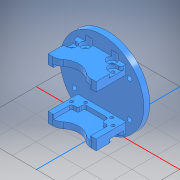
# Autodesk Inventor part: 000.005.005.001 - Основание
Saved by Autodesk Inventor 2022 (Build 260153000, 153)
## iProperties
Created: 2022-12-19
Part Number: 000.005.005.001 - Основание
Material: Пластик АБС
Document SubType Name: Modeling
Designer: Ivan Petrov
Density: 1.06 g/cm^3
Appearance: Голубой
Author: Ivan Petrov
Autodesk Inventor part; units mm, degrees
ref_plane "YZ Plane" through (0, 0, 0) normal (1, 0, 0) x (0, 1, 0)
ref_plane "XZ Plane" through (0, 0, 0) normal (0, 1, 0) x (-1, 0, 0)
ref_plane "XY Plane" through (0, 0, 0) normal (0, 0, 1) x (1, 0, 0)
sketch "Эскиз1" plane through (0, 0, 0) normal (0, 0, 1) x (1, 0, 0)
  circle A0 centre (0, 0) radius 35
  dimension "d7" = 70
  constraints: 1 centre point
  measures "d7" diameter of A0
extrude "Выдавливание1" add sketch "Эскиз1" along normal blind 5
sketch "Эскиз2" plane through (0, 0, 5) normal (0, 0, 1) x (1, 0, 0)
  circle A0 centre (-23, 15) radius 2
  point P0 (0, 0)
  dimension "d4" = 4
  dimension "d5" = 15
  dimension "d6" = 23
  constraints: 1 centre point
  measures "d4" diameter of A0
  measures "d5" vertical distance of A0.centre point (0, 0)
  measures "d6" horizontal distance of point (0, 0) A0.centre
extrude "Выдавливание2" cut sketch "Эскиз2" against normal through all
mirror "Зеркальное отражение1" about plane through (0, 0, 0) normal (0, 1, 0) of "Выдавливание2"
mirror "Зеркальное отражение2" about plane through (0, 0, 0) normal (1, 0, 0) of "Выдавливание2", "Зеркальное отражение1"
sketch "Эскиз9" plane through (0, 0, 5) normal (0, 0, 1) x (1, 0, 0)
  line L0 (20.1, 16) -> (20.1, 13.5) projected
  line L1 (-20.1, 16) -> (-20.1, 13.5) projected
  line L2 (20.1, 16) -> (-20.1, 16)
  line L3 (-20.1, 16) -> (-20.1, 18.6)
  line L4 (-20.1, 18.6) -> (20.1, 18.6)
  line L5 (20.1, 18.6) -> (20.1, 16)
  line L6 (-13, 18.6) -> (13, 18.6)
  point P0 (0, 0)
  constraints: 10 end point, 2 horizontal, 2 parallel, 1 perpendicular, 1 point on line, 2 other
extrude "Выдавливание8" add sketch "Эскиз9" along normal blind 25
sketch "Эскиз10" plane through (0, 0, 5) normal (0, 0, 1) x (1, 0, 0)
  line L0 (20.1, -15.5) -> (20.1, -18) projected
  line L1 (-20.1, -15.5) -> (-20.1, -18) projected
  line L2 (20.1, -18) -> (-20.1, -18)
  line L3 (-20.1, -18) -> (-20.1, -21.5)
  line L4 (-20.1, -21.5) -> (20.1, -21.5)
  line L5 (20.1, -21.5) -> (20.1, -18)
  line L6 (7.6826, -21.5) -> (-7.6826, -21.5) projected
  point P0 (0, 0)
  constraints: 8 end point, 2 parallel, 1 horizontal, 1 perpendicular, 1 point on line
extrude "Выдавливание9" add sketch "Эскиз10" along normal blind 25
sketch "Эскиз11" plane through (-20.1, 18.6, 5) normal (0, 1, 0) x (1, 0, 0)
  arc A0 (0, -52.6766) -> (0.5192, -54.3636) centre (3, -52.6766) ccw
  line L0 (0.5192, -54.3636) -> (4.5047, -60.2246)
  arc A1 (4.5047, -60.2246) -> (6.1586, -61.1) centre (6.1586, -59.1) ccw
  line L1 (7.1, -61.1) -> (6.1586, -61.1)
  arc A2 (5.6, -59.6) -> (7.1, -61.1) centre (7.1, -59.6) ccw
  line L2 (5.6, -6.6) -> (5.6, -59.6)
  arc A3 (6.6, -5.6) -> (5.6, -6.6) centre (6.6, -6.6) ccw
  line L3 (33.6, -5.6) -> (6.6, -5.6)
  arc A4 (34.6, -6.6) -> (33.6, -5.6) centre (33.6, -6.6) ccw
  line L4 (34.6, -59.6) -> (34.6, -6.6)
  arc A5 (33.1, -61.1) -> (34.6, -59.6) centre (33.1, -59.6) ccw
  line L5 (34.0414, -61.1) -> (33.1, -61.1)
  arc A6 (34.0414, -61.1) -> (35.6953, -60.2246) centre (34.0414, -59.1) ccw
  line L6 (35.6953, -60.2246) -> (39.6808, -54.3636)
  arc A7 (39.6808, -54.3636) -> (40.2, -52.6766) centre (37.2, -52.6766) ccw
  line L7 (40.2, -52.6766) -> (40.2, -8.4234)
  arc A8 (40.2, -8.4234) -> (39.6808, -6.7364) centre (37.2, -8.4234) ccw
  line L8 (39.6808, -6.7364) -> (35.9929, -1.3131)
  arc A9 (35.9929, -1.3131) -> (33.5121, 0) centre (33.5121, -3) ccw
  line L9 (33.5121, 0) -> (6.6879, 0)
  arc A10 (6.6879, 0) -> (4.2071, -1.3131) centre (6.6879, -3) ccw
  line L10 (4.2071, -1.3131) -> (0.5192, -6.7364)
  arc A11 (0.5192, -6.7364) -> (0, -8.4234) centre (3, -8.4234) ccw
  line L11 (0, -8.4234) -> (0, -52.6766)
  circle A12 centre (37.4, -52.1) radius 1.35
  circle A13 centre (37.4, -30.1) radius 1.35
  circle A14 centre (31.1, -2.8) radius 1.35
  circle A15 centre (2.8, -52.1) radius 1.35
  circle A16 centre (2.8, -30.1) radius 1.35
  circle A17 centre (9.1, -2.8) radius 1.35
  circle A18 centre (37.4, -8.1) radius 1.35
  circle A19 centre (2.8, -8.1) radius 1.35
  line L12 (7.1, -61.1) -> (33.1, -61.1)
  point P0 (20.1, 5)
  point P1 (20.1, -48.1)
  point P2 (20.1, -48.1)
  constraints: 26 end point, 24 point on circle, 20 centre point
extrude "Выдавливание10" cut sketch "Эскиз11" against normal through all contours A14 | A17 | A18 | A19
sketch "Эскиз12" plane through (-20.1, 18.6, 5) normal (0, 1, 0) x (1, 0, 0)
  arc A0 (0, -52.6766) -> (0.5192, -54.3636) centre (3, -52.6766) ccw
  line L0 (0.5192, -54.3636) -> (4.5047, -60.2246)
  arc A1 (4.5047, -60.2246) -> (6.1586, -61.1) centre (6.1586, -59.1) ccw
  line L1 (7.1, -61.1) -> (6.1586, -61.1)
  arc A2 (5.6, -59.6) -> (7.1, -61.1) centre (7.1, -59.6) ccw
  line L2 (5.6, -6.6) -> (5.6, -59.6)
  arc A3 (6.6, -5.6) -> (5.6, -6.6) centre (6.6, -6.6) ccw
  line L3 (33.6, -5.6) -> (6.6, -5.6)
  arc A4 (34.6, -6.6) -> (33.6, -5.6) centre (33.6, -6.6) ccw
  line L4 (34.6, -59.6) -> (34.6, -6.6)
  arc A5 (33.1, -61.1) -> (34.6, -59.6) centre (33.1, -59.6) ccw
  line L5 (34.0414, -61.1) -> (33.1, -61.1)
  arc A6 (34.0414, -61.1) -> (35.6953, -60.2246) centre (34.0414, -59.1) ccw
  line L6 (35.6953, -60.2246) -> (39.6808, -54.3636)
  arc A7 (39.6808, -54.3636) -> (40.2, -52.6766) centre (37.2, -52.6766) ccw
  line L7 (40.2, -52.6766) -> (40.2, -8.4234)
  arc A8 (40.2, -8.4234) -> (39.6808, -6.7364) centre (37.2, -8.4234) ccw
  line L8 (39.6808, -6.7364) -> (35.9929, -1.3131)
  arc A9 (35.9929, -1.3131) -> (33.5121, 0) centre (33.5121, -3) ccw
  line L9 (33.5121, 0) -> (6.6879, 0)
  arc A10 (6.6879, 0) -> (4.2071, -1.3131) centre (6.6879, -3) ccw
  line L10 (4.2071, -1.3131) -> (0.5192, -6.7364)
  arc A11 (0.5192, -6.7364) -> (0, -8.4234) centre (3, -8.4234) ccw
  line L11 (0, -8.4234) -> (0, -52.6766)
  circle A12 centre (37.4, -52.1) radius 1.35
  circle A13 centre (37.4, -30.1) radius 1.35
  circle A14 centre (31.1, -2.8) radius 1.35
  circle A15 centre (2.8, -52.1) radius 1.35
  circle A16 centre (2.8, -30.1) radius 1.35
  circle A17 centre (9.1, -2.8) radius 1.35
  circle A18 centre (37.4, -8.1) radius 1.35
  circle A19 centre (2.8, -8.1) radius 1.35
  line L12 (7.1, -61.1) -> (33.1, -61.1)
  point P0 (20.1, 5)
  point P1 (20.1, 5)
  point P2 (20.1, -48.1)
  point P3 (20.1, -48.1)
  constraints: 26 end point, 24 point on circle, 20 centre point
extrude "Выдавливание11" cut sketch "Эскиз12" against normal blind 10 contours A2 L2 A3 L3 A4 L4 A5 L12
sketch "Эскиз13" plane through (-20.1, -21.5, 5) normal (0, -1, 0) x (1, 0, 0)
  arc A0 (0.5192, 54.3636) -> (0, 52.6766) centre (3, 52.6766) ccw
  line L0 (0, 8.4234) -> (0, 52.6766)
  arc A1 (0, 8.4234) -> (0.5192, 6.7364) centre (3, 8.4234) ccw
  line L1 (4.2071, 1.3131) -> (0.5192, 6.7364)
  arc A2 (4.2071, 1.3131) -> (6.6879, 0) centre (6.6879, 3) ccw
  line L2 (33.5121, 0) -> (6.6879, 0)
  arc A3 (33.5121, 0) -> (35.9929, 1.3131) centre (33.5121, 3) ccw
  line L3 (39.6808, 6.7364) -> (35.9929, 1.3131)
  arc A4 (39.6808, 6.7364) -> (40.2, 8.4234) centre (37.2, 8.4234) ccw
  line L4 (40.2, 52.6766) -> (40.2, 8.4234)
  arc A5 (40.2, 52.6766) -> (39.6808, 54.3636) centre (37.2, 52.6766) ccw
  line L5 (35.6953, 60.2246) -> (39.6808, 54.3636)
  arc A6 (35.6953, 60.2246) -> (34.0414, 61.1) centre (34.0414, 59.1) ccw
  line L6 (27.75, 61.1) -> (34.0414, 61.1)
  arc A7 (29.25, 59.6) -> (27.75, 61.1) centre (27.75, 59.6) ccw
  line L7 (29.25, 59.6) -> (29.25, 58.1)
  arc A8 (29.25, 58.1) -> (31.6, 55.75) centre (31.6, 58.1) ccw
  line L8 (31.6, 55.75) -> (33.6, 55.75)
  arc A9 (34.6, 54.75) -> (33.6, 55.75) centre (33.6, 54.75) ccw
  line L9 (34.6, 54.75) -> (34.6, 11.95)
  arc A10 (33.6, 10.95) -> (34.6, 11.95) centre (33.6, 11.95) ccw
  line L10 (33.6, 10.95) -> (31.6, 10.95)
  arc A11 (31.6, 10.95) -> (29.25, 8.6) centre (31.6, 8.6) ccw
  line L11 (29.25, 8.6) -> (29.25, 6.6)
  arc A12 (28.25, 5.6) -> (29.25, 6.6) centre (28.25, 6.6) ccw
  line L12 (28.25, 5.6) -> (11.95, 5.6)
  arc A13 (10.95, 6.6) -> (11.95, 5.6) centre (11.95, 6.6) ccw
  line L13 (10.95, 6.6) -> (10.95, 8.6)
  arc A14 (10.95, 8.6) -> (8.6, 10.95) centre (8.6, 8.6) ccw
  line L14 (8.6, 10.95) -> (6.6, 10.95)
  arc A15 (5.6, 11.95) -> (6.6, 10.95) centre (6.6, 11.95) ccw
  line L15 (5.6, 11.95) -> (5.6, 54.75)
  arc A16 (6.6, 55.75) -> (5.6, 54.75) centre (6.6, 54.75) ccw
  line L16 (6.6, 55.75) -> (8.6, 55.75)
  arc A17 (8.6, 55.75) -> (10.95, 58.1) centre (8.6, 58.1) ccw
  line L17 (10.95, 58.1) -> (10.95, 59.6)
  arc A18 (12.45, 61.1) -> (10.95, 59.6) centre (12.45, 59.6) ccw
  line L18 (6.1586, 61.1) -> (12.45, 61.1)
  arc A19 (6.1586, 61.1) -> (4.5047, 60.2246) centre (6.1586, 59.1) ccw
  line L19 (0.5192, 54.3636) -> (4.5047, 60.2246)
  circle A20 centre (37.4, 52.1) radius 1.35
  circle A21 centre (37.4, 30.1) radius 1.35
  circle A22 centre (31.1, 2.8) radius 1.35
  circle A23 centre (2.8, 52.1) radius 1.35
  circle A24 centre (2.8, 30.1) radius 1.35
  circle A25 centre (9.1, 2.8) radius 1.35
  circle A26 centre (37.4, 8.1) radius 1.35
  circle A27 centre (2.8, 8.1) radius 1.35
  circle A28 centre (20.1, 48.1) radius 1.6 projected
  line L20 (12.45, 61.1) -> (27.75, 61.1)
  point P0 (20.1, -5)
  constraints: 42 end point, 40 point on circle, 28 centre point, 1 horizontal
extrude "Выдавливание12" cut sketch "Эскиз13" against normal blind 10 contours L20 A7 L7 A8 L8 A9 L9 A10 L10 A11 L11 A12 L12 A13 L13 A14 L14 A15 L15 A16 L16 A17 L17 A18
offset faces "Размер5" outward -1 faces at (-14.5, 17.7333, 17.7333) (-14.4556, 17.7333, 11.3052) (4.5, 17.7333, 10.6) (14.4309, 16.8667, 11.2347) (14.5, 17.7333, 23.8667) (-2.7167, -20.3333, 10.6) (8.2247, -20.3333, 10.6028) (9.1762, -19.1667, 13.9502) (9.15, -20.3333, 12.2667) (12.1667, -20.3333, 15.95) (14.4888, -19.1667, 16.801) (14.5, -19.1667, 21.3) (-9.1388, -19.1667, 11.451) (-9.15, -20.3333, 12.9333) (-11.1498, -19.1667, 15.9238) (-12.8333, -19.1667, 15.95) (-14.1802, -19.1667, 16.2169) (-14.5, -20.3333, 25.65)
sketch "Эскиз14" plane through (-20.1, -21.5, 5) normal (0, -1, 0) x (1, 0, 0)
  line L0 (35.6, 25) -> (35.6, 11.95) projected
  arc A0 (33.6, 9.95) -> (35.6, 11.95) centre (33.6, 11.95) ccw projected
  line L1 (33.6, 9.95) -> (31.6, 9.95) projected
  arc A1 (31.6, 9.95) -> (30.25, 8.6) centre (31.6, 8.6) ccw projected
  line L2 (30.25, 8.6) -> (30.25, 6.6) projected
  arc A2 (28.25, 4.6) -> (30.25, 6.6) centre (28.25, 6.6) ccw projected
  line L3 (28.25, 4.6) -> (11.95, 4.6) projected
  arc A3 (9.95, 6.6) -> (11.95, 4.6) centre (11.95, 6.6) ccw projected
  line L4 (9.95, 6.6) -> (9.95, 8.6) projected
  arc A4 (9.95, 8.6) -> (8.6, 9.95) centre (8.6, 8.6) ccw projected
  line L5 (8.6, 9.95) -> (6.6, 9.95) projected
  arc A5 (4.6, 11.95) -> (6.6, 9.95) centre (6.6, 11.95) ccw projected
  line L6 (4.6, 11.95) -> (4.6, 25) projected
  line L7 (0, 25) -> (4.6, 25) projected
  line L8 (0, 0) -> (0, 25) projected
  line L9 (40.2, 0) -> (0, 0) projected
  line L10 (40.2, 0) -> (40.2, 25) projected
  line L11 (35.6, 25) -> (40.2, 25) projected
  circle A6 centre (37.4, 8.1) radius 1.35 projected
  circle A7 centre (2.8, 8.1) radius 1.35 projected
  circle A8 centre (31.1, 2.8) radius 1.35 projected
  circle A9 centre (9.1, 2.8) radius 1.35 projected
  line L12 (4.6, 6.6) -> (4.6, 25) projected
  line L13 (4.6, 25) -> (36.05, 25)
  point P0 (20.1, -5)
  constraints: 2 end point, 1 point on line
extrude "Выдавливание13" add sketch "Эскиз14" along normal blind 5
sketch "Эскиз15" plane through (-20.1, 18.6, 5) normal (0, 1, 0) x (1, 0, 0)
  line L0 (4.6, -25) -> (4.6, -6.6) projected
  arc A0 (6.6, -4.6) -> (4.6, -6.6) centre (6.6, -6.6) ccw projected
  line L1 (6.6, -4.6) -> (33.6, -4.6) projected
  arc A1 (35.6, -6.6) -> (33.6, -4.6) centre (33.6, -6.6) ccw projected
  line L2 (35.6, -6.6) -> (35.6, -25) projected
  line L3 (40.2, -25) -> (35.6, -25) projected
  line L4 (40.2, 0) -> (40.2, -25) projected
  line L5 (0, 0) -> (40.2, 0) projected
  line L6 (0, 0) -> (0, -25) projected
  line L7 (4.6, -25) -> (0, -25) projected
  circle A2 centre (37.4, -8.1) radius 1.35 projected
  circle A3 centre (2.8, -8.1) radius 1.35 projected
  circle A4 centre (31.1, -2.8) radius 1.35 projected
  circle A5 centre (9.1, -2.8) radius 1.35 projected
  line L8 (35.6, -25) -> (4.6, -25)
  line L9 (40.2, -25) -> (0, -25) projected
  point P0 (20.1, 5)
  constraints: 2 end point, 1 collinear
extrude "Выдавливание14" add sketch "Эскиз15" along normal blind 5
sketch "Эскиз16" plane through (-20.1, 23.6, 5) normal (0, 1, 0) x (1, 0, 0)
  circle A0 centre (37.4, -8.1) radius 1.35 projected
  circle A1 centre (37.4, -8.1) radius 4
  circle A2 centre (31.1, -2.8) radius 1.35 projected
  circle A3 centre (31.1, -2.8) radius 4
  circle A4 centre (2.8, -8.1) radius 1.35 projected
  circle A5 centre (2.8, -8.1) radius 4
  circle A6 centre (9.1, -2.8) radius 1.35 projected
  circle A7 centre (9.1, -2.8) radius 4
  point P0 (20.1, 5)
  dimension "d51" = 8
  dimension "d52" = 8
  dimension "d53" = 8
  dimension "d54" = 8
  constraints: 4 centre point, 4 coincident
  measures "d51" diameter of A1
  measures "d52" diameter of A3
  measures "d53" diameter of A5
  measures "d54" diameter of A7
extrude "Выдавливание15" cut sketch "Эскиз16" along normal blind 4.5 and the other way blind 3 contours A0 | A1 | A2 | A3 | A4 | A5 | A6 | A7
fillet "Сопряжение3" radius 2 4 edges at (20.1, 22.1, 15.9566) (20.1, 22.1, 10.2434) (-20.1, 22.1, 15.9566) (-20.1, 22.1, 10.2434)
sketch "Эскиз17" plane through (-20.1, -26.5, 5) normal (0, -1, 0) x (1, 0, 0)
  circle A0 centre (2.8, 8.1) radius 1.35 projected
  circle A1 centre (2.8, 8.1) radius 4
  circle A2 centre (9.1, 2.8) radius 1.35 projected
  circle A3 centre (9.1, 2.8) radius 4
  circle A4 centre (31.1, 2.8) radius 1.35 projected
  circle A5 centre (31.1, 2.8) radius 4
  circle A6 centre (37.4, 8.1) radius 1.35 projected
  circle A7 centre (37.4, 8.1) radius 4
  point P0 (20.1, -5)
  dimension "d60" = 8
  dimension "d61" = 8
  dimension "d62" = 8
  dimension "d63" = 8
  constraints: 4 centre point, 4 coincident
  measures "d60" diameter of A1
  measures "d61" diameter of A3
  measures "d62" diameter of A5
  measures "d63" diameter of A7
extrude "Выдавливание16" cut sketch "Эскиз17" along normal blind 4.5 and the other way blind 3 contours A0 | A1 | A2 | A3 | A4 | A5 | A6 | A7
fillet "Сопряжение4" radius 2 4 edges at (20.1, -25, 15.9566) (20.1, -25, 10.2434) (-20.1, -25, 10.2434) (-20.1, -25, 15.9566)
sketch "Эскиз18" plane through (-20.1, 23.6, 5) normal (0, 1, 0) x (1, 0, 0)
  line L0 (35.6, -25) -> (4.6, -25) projected
  arc A0 (31.9916, -25) -> (8.2084, -25) centre (20.1, -34.5388) ccw
  line L1 (20.1, 5) -> (20.1, -9.2015) construction
  constraints: 2 end point, 2 point on circle, 2 point on line, 1 centre point, 1 symmetric about line, 1 vertical, 1 vertical alignment
extrude "Выдавливание17" cut sketch "Эскиз18" against normal through all
fillet "Сопряжение5" radius 10.75 4 edges at (-11.8916, 21.1, 30) (11.8916, 21.1, 30) (-11.8916, -24, 30) (11.8916, -24, 30)
